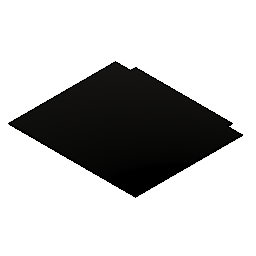
z-stage_assembly_2 v13 (Autodesk Fusion 360 archive; units mm, degrees)
design "Magnetic_224x254_sheet"
Autodesk Fusion 360 part; units mm, degrees
sketch "Sketch1" plane through (0, 0, 0) normal (0, 0, 1) x (1, 0, 0)
  line L0 (127, -112) -> (-127, -112)
  line L1 (-127, -112) -> (-127, 112)
  line L2 (-127, 112) -> (127, 112)
  line L3 (127, 112) -> (127, -112)
  line L4 (127, -112) -> (-127, 112) construction
  line L5 (-127, -112) -> (127, 112) construction
  dimension "d1" = 254
  dimension "d2" = 224
  constraint perpendicular L0 L1
  constraint parallel L0 L2
  constraint parallel L1 L3
  constraint horizontal L0
  constraint coincident L4 origin
  constraint coincident L5 origin
  measures "d1" distance of L1.end L2.end
  measures "d2" distance of L0.start L2.end
extrude "Extrude1" add sketch "Sketch1" along normal blind 1.36
sketch "Sketch2" plane through (0, 0, 1.36) normal (0, 0, 1) x (-1, 0, 0)
  line L0 (-127, -112) -> (127, -112)
  line L1 (127, -112) -> (127, 112)
  line L2 (127, 112) -> (-127, 112)
  line L3 (-127, 112) -> (-127, -112)
  line L4 (-127, 98) -> (-113, 112)
  dimension "d5" = 45
  dimension "d6" = 14
  constraint coincident L3 L4.start
  constraint coincident L2 L4.end
  measures "d5" angle of L2 L4
  measures "d6" distance of L2 L4.start
extrude "Extrude2" [suppressed]
mirror "Mirror1" [suppressed]
sketch "Sketch3" plane through (0, 0, 1.36) normal (0, 0, 1) x (-1, 0, 0)
  line L0 (127, 112) -> (-127, 112)
  line L1 (-127, 112) -> (-127, -112)
  line L2 (-127, -112) -> (127, -112)
  line L3 (127, -112) -> (127, 112)
  line L4 (127, -112) -> (97, -112)
  line L5 (97, -112) -> (97, -102)
  line L6 (97, -102) -> (127, -102)
  line L7 (127, -102) -> (127, -112)
  dimension "d9" = 30
  dimension "d10" = 10
  constraint horizontal L4
  constraint vertical L5
  constraint horizontal L6
  constraint vertical L7
  constraint coincident L2.end L3.start
  measures "d9" distance of L2.end L4.end
  measures "d10" distance of L2.end L6.end
extrude "Extrude3" cut sketch "Sketch3" against normal through all contours L2 L3 L4 L5 L6 L7
mirror "Mirror2" about plane through (0, 0, 0) normal (1, 0, 0) of "Extrude3"

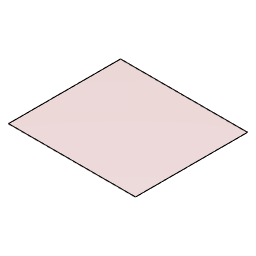
design "PEI_224x254_sheet"
Autodesk Fusion 360 part; units mm, degrees
sketch "Sketch1" plane through (0, 0, 0) normal (0, 0, 1) x (1, 0, 0)
  line L0 (127, -112) -> (-127, -112)
  line L1 (-127, -112) -> (-127, 112)
  line L2 (-127, 112) -> (127, 112)
  line L3 (127, 112) -> (127, -112)
  line L4 (127, -112) -> (-127, 112) construction
  line L5 (-127, -112) -> (127, 112) construction
  dimension "d1" = 254
  dimension "d2" = 224
  constraint perpendicular L0 L1
  constraint parallel L0 L2
  constraint parallel L1 L3
  constraint horizontal L0
  constraint coincident L4 origin
  constraint coincident L5 origin
  measures "d1" distance of L1.end L2.end
  measures "d2" distance of L0.start L2.end
extrude "Extrude1" add sketch "Sketch1" along normal blind 0.2
sketch "Sketch2" plane through (0, 0, 0.2) normal (0, 0, 1) x (-1, 0, 0)
  line L0 (-127, -112) -> (127, -112)
  line L1 (127, -112) -> (127, 112)
  line L2 (127, 112) -> (-127, 112)
  line L3 (-127, 112) -> (-127, -112)
sketch "Sketch3" plane through (0, 0, 0.2) normal (0, 0, 1) x (-1, 0, 0)
  line L0 (127, 112) -> (-127, 112) construction
  line L1 (-127, -112) -> (127, -112) construction
  line L2 (-97, 112) -> (-97, -112) construction
  line L3 (-127, 112) -> (-127, -112) construction
  line L4 (127, -112) -> (127, 112) construction
  line L5 (-127, -107) -> (127, -107) construction
  line L6 (-97, -107) -> (103, -107) construction
  line L7 (103, -107) -> (103, 103) construction
  line L8 (103, 103) -> (-97, 103) construction
  line L9 (-97, 103) -> (-97, -107) construction
  line L10 (103, 103) -> (-97, -107) construction
  line L11 (-97, 103) -> (103, -107) construction
  point P0 (3, -2)
  dimension "d5" = 30
  dimension "d6" = 5
  dimension "d7" = 200
  dimension "d8" = 210
  constraint coincident L0 L2.start
  constraint coincident L1 L2.end
  constraint perpendicular L1 L2
  constraint coincident L3 L5.start
  constraint coincident L4 L5.end
  constraint perpendicular L3 L5
  constraint horizontal L6
  constraint vertical L7
  constraint horizontal L8
  constraint vertical L9
  constraint coincident L2 L6.start
  constraint coincident L5 L6.start
  constraint midpoint L10 P0
  measures "d5" distance of L2 L3
  measures "d6" distance of L1 L5
  measures "d7" distance of L7.end L8.end
  measures "d8" distance of L6.end L7.end
sketch "Sketch4" plane through (0, 0, 0.2) normal (0, 0, 1) x (-1, 0, 0)
  line L0 (-127, -112) -> (127, -112) construction
  line L1 (127, 112) -> (-127, 112) construction
  line L2 (97, -112) -> (97, 112) construction
  line L3 (127, -112) -> (127, 112) construction
  line L4 (-127, 112) -> (-127, -112) construction
  line L5 (127, 100) -> (-127, 100) construction
  line L6 (97, 100) -> (-103, 100) construction
  line L7 (-103, 100) -> (-103, -108) construction
  line L8 (-103, -108) -> (97, -108) construction
  line L9 (97, -108) -> (97, 100) construction
  line L10 (97, -108) -> (-103, 100) construction
  line L11 (-103, -108) -> (97, 100) construction
  point P0 (-3, -4)
  dimension "d9" = 30
  dimension "d10" = 12
  dimension "d11" = 200
  dimension "d12" = 208
  constraint coincident L0 L2.start
  constraint coincident L1 L2.end
  constraint perpendicular L1 L2
  constraint coincident L3 L5.start
  constraint coincident L4 L5.end
  constraint perpendicular L3 L5
  constraint horizontal L6
  constraint vertical L7
  constraint horizontal L8
  constraint vertical L9
  constraint coincident L2 L6.start
  constraint coincident L5 L6.start
  constraint midpoint L11 P0
  measures "d9" distance of L2 L3
  measures "d10" distance of L1 L5
  measures "d11" distance of L7.end L8.end
  measures "d12" distance of L6.end L7.end

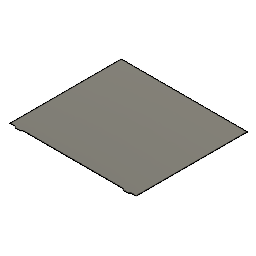
design "Spring_Steel_224x254_sheet"
Autodesk Fusion 360 part; units mm, degrees
sketch "Sketch1" plane through (0, 0, 0) normal (0, 0, 1) x (1, 0, 0)
  line L0 (127, -112) -> (-127, -112)
  line L1 (-127, -112) -> (-127, 112)
  line L2 (-127, 112) -> (127, 112)
  line L3 (127, 112) -> (127, -112)
  line L4 (127, -112) -> (-127, 112) construction
  line L5 (-127, -112) -> (127, 112) construction
  dimension "d1" = 254
  dimension "d2" = 224
  constraint perpendicular L0 L1
  constraint parallel L0 L2
  constraint parallel L1 L3
  constraint horizontal L0
  constraint coincident L4 origin
  constraint coincident L5 origin
  measures "d1" distance of L1.end L2.end
  measures "d2" distance of L0.start L2.end
extrude "Extrude1" add sketch "Sketch1" along normal blind 0.5
sketch "Sketch3" plane through (0, 0, 0.5) normal (0, 0, 1) x (-1, 0, 0)
  line L0 (127, 112) -> (-127, 112)
  line L1 (-127, 112) -> (-127, -112)
  line L2 (-127, -112) -> (127, -112)
  line L3 (127, -112) -> (127, 112)
  line L4 (116.4, 112) -> (113.52, 114.88)
  line L5 (113.52, 114.88) -> (103.32, 114.88)
  line L6 (103.32, 114.88) -> (100.44, 112)
  line L7 (0, 0) -> (0, -112) construction
  line L8 (-116.4, 112) -> (-113.52, 114.88)
  line L9 (-113.52, 114.88) -> (-103.32, 114.88)
  line L10 (-103.32, 114.88) -> (-100.44, 112)
  dimension "d13" = 10.6
  dimension "d14" = 10.2
  constraint coincident L7.start origin
  constraint midpoint L2 L7.end
  constraint symmetric L4.start L7 L8.start
  constraint symmetric L4.end L7 L8.end
  constraint symmetric L5.end L7 L9.end
  constraint symmetric L6.end L7 L10.end
  measures "d13" distance of L3 L4.start
  measures "d14" distance of L4.end L5.end
extrude "Extrude3" add sketch "Sketch3" against normal up to surface (0.5 mm away) contours L0 L4 L5 L6 | L0 L8 L9 L10
fillet "Fillet2" radius 1 4 edges at (-100.44, -112, 0.25) (-103.32, -114.88, 0.25) (-113.52, -114.88, 0.25) (-116.4, -112, 0.25)
fillet "Fillet2" radius 1 4 edges at (116.4, -112, 0.25) (113.52, -114.88, 0.25) (103.32, -114.88, 0.25) (100.44, -112, 0.25)
